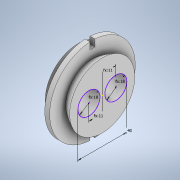
# Autodesk Inventor part: SpacerCorrect
Saved by Autodesk Inventor 2021.2 (Build 252289000, 289)
## iProperties
Created: 2023-01-30
Part Number: SpacerCorrect
Material: Типовые
Document SubType Name: Modeling
Designer: Andrei
Density: 1 g/cm^3
Appearance: По умолчанию
Author: Andrei
Autodesk Inventor part; units mm, degrees
ref_plane "YZ Plane" through (0, 0, 0) normal (1, 0, 0) x (0, 1, 0)
ref_plane "XZ Plane" through (0, 0, 0) normal (0, 1, 0) x (-1, 0, 0)
ref_plane "XY Plane" through (0, 0, 0) normal (0, 0, 1) x (1, 0, 0)
sketch "Эскиз1" plane through (0, 0, 0) normal (0, 0, 1) x (1, 0, 0)
  line L0 (0, 0) -> (2, 0)
  line L1 (2, 0) -> (2, -35)
  line L2 (2, -35) -> (0, -35)
  line L3 (0, -35) -> (0, 0)
  line L4 (2, 0) -> (10, 0)
  line L5 (10, 0) -> (10, -26.6188)
  line L6 (10, -26.6188) -> (2, -26.6188)
  line L7 (2, -26.6188) -> (2, 0)
  line L8 (2, 0) -> (2, -22)
  line L9 (2, -22) -> (10, -26.6188)
  dimension "d0" = 2
  dimension "d1" = 35
  dimension "d2" = 8
  dimension "d4" = 22
  dimension "d36" = 60
  constraints: 20 end point, 4 parallel, 2 horizontal, 2 perpendicular, 1 point on line
  measures "d0" distance of L1.end L2.end
  measures "d1" distance of L0.end L1.end
  measures "d2" distance of L5.end L6.end
  measures "d4" distance of L0.end L8.end
  measures "d36" angle of L9 L1
revolve "Вращение1" add sketch "Эскиз1" angle 360 about axis through (0, 0, 0) along (1, 0, 0) contours L0 L1 L2 L3 | L4 L5 L9 L1
mirror "Зеркальное отражение1" about plane through (0, 0, 0) normal (-1, 0, 0)
sketch "Эскиз2" plane through (10, 0, 0) normal (1, 0, 0) x (0, 0, -1)
  circle A0 centre (11, 0) radius 9
  circle A1 centre (-11, 0) radius 9
  point P0 (0, 0)
  dimension "d6" = 18
  dimension "d7" = 18
  dimension "d8" = 11
  dimension "d9" = 11
  dimension "d10" = 40
  constraints: 2 centre point
  measures "d6" diameter of A0
  measures "d7" diameter of A1
  measures "d8" distance of A0.centre point (0, 0)
  measures "d9" distance of A1.centre point (0, 0)
hole "Отверстие1" at (10, 0, 11) direction (-1, 0, 0) diameter 18 end through all
hole "Отверстие2" at (10, 0, -11) direction (-1, 0, 0) diameter 18 end through all
sketch "Эскиз3" plane through (2, 0, 0) normal (1, 0, 0) x (0, 0, -1)
  line L0 (-2, 35) -> (2, 35)
  line L1 (2, 35) -> (2, 29.3705)
  line L2 (2, 29.3705) -> (-2, 29.3705)
  line L3 (-2, 29.3705) -> (-2, 35)
  circle A0 centre (0, 0) radius 35 projected
  line L4 (0, 35) -> (0, 29)
  line L5 (0, -35) -> (0, -29)
  line L6 (-2, -29) -> (2, -29)
  line L7 (2, -29) -> (2, -35)
  line L8 (2, -35) -> (-2, -35)
  line L9 (-2, -35) -> (-2, -29)
  dimension "d25" = 4
  dimension "d26" = 6
  dimension "d27" = 2
  dimension "d28" = 0
  dimension "d29" = 6
  dimension "d30" = 6
  dimension "d31" = 4
  dimension "d32" = 2
  dimension "d33" = 0
  constraints: 20 end point, 4 parallel, 2 horizontal, 2 perpendicular, 2 point on circle, 2 vertical
  measures "d25" distance of L1.end L2.end
  measures "d26" distance of L4.start L4.end
  measures "d27" distance between parallel lines of L4 L3
  measures "d28" distance from line of L4.start L0
  measures "d29" distance of L5.start L5.end
  measures "d30" distance of L6.end L7.end
  measures "d31" distance of L6.start L6.end
  measures "d32" distance between parallel lines of L5 L9
  measures "d33" distance from line of L5.end L6
extrude "Выдавливание1" cut sketch "Эскиз3" against normal through all contours L0 A0 L3 | L0 L1 A0 | L4 L2 L3 A0 | A0 L1 L2 L4 | L9 L6 L5 A0 | A0 L8 L9 | L5 L6 L7 A0 | A0 L7 L8
equation "\"d0\" = 0.5 * hFlange"
equation "\"d1\" = 0.5 * dOuter"
equation "\"d2\" = hMount"
equation "\"d4\" = 0.5 * dMinimal"
equation "\"d36\" = angleMount"
equation "\"d6\" = dHoles"
equation "\"d7\" = dHoles"
equation "\"d8\" = r2holes"
equation "\"d9\" = r2holes"
equation "\"d11\" = dHoles"
equation "\"d18\" = dHoles"
equation "\"d25\" = wSlot"
equation "\"d26\" = hSlot"
equation "\"d27\" = 0.5 * wSlot"
equation "\"d29\" = hSlot"
equation "\"d30\" = hSlot"
equation "\"d31\" = wSlot"
equation "\"d32\" = 0.5 * wSlot"
equation "\"hFlange\" = 4"
equation "\"dMinimal\" = 44"
equation "\"angleMount\" = 60deg"
equation "\"dHoles\" = 18"
equation "\"r2holes\" = 11"
equation "\"hMount\" = 8"
equation "\"wSlot\" = 4"
equation "\"hSlot\" = 6"
equation "\"dOuter\" = 70"
